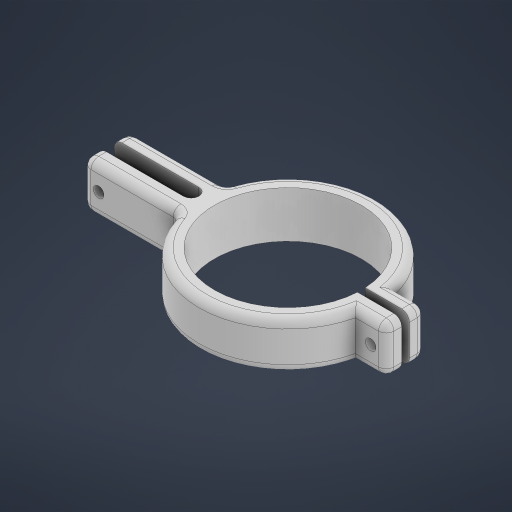
# Autodesk Inventor part: Clamp
Saved by Autodesk Inventor 2024.1 (Build 281209000, 209)
## iProperties
Created: 2024-11-18
Part Number: Clamp
Material: Generic
Document SubType Name: Modeling
Designer: Designer
Density: 1 g/cm^3
Appearance: Default
Author: Designer
Autodesk Inventor part; units mm, degrees
ref_plane "YZ Plane" through (0, 0, 0) normal (1, 0, 0) x (0, 1, 0)
ref_plane "XZ Plane" through (0, 0, 0) normal (0, 1, 0) x (-1, 0, 0)
ref_plane "XY Plane" through (0, 0, 0) normal (0, 0, 1) x (1, 0, 0)
sketch "Sketch1" plane through (0, 0, 0) normal (0, 1, 0) x (-1, 0, 0)
  line L0 (-22.0113, 1.5875) -> (-22.0113, 7.9375)
  line L1 (-22.0113, 7.9375) -> (-9.3113, 7.9375)
  arc A0 (-3.8366, -1.5875) -> (-3.8366, 1.5875) centre (26.2841, 0) ccw
  line L2 (-22.0113, 1.5875) -> (-8.3646, 1.5875)
  line L3 (-8.3646, -1.5875) -> (-22.0113, -1.5875)
  line L4 (-22.0113, -1.5875) -> (-22.0113, -7.9375)
  line L5 (-22.0113, -7.9375) -> (-9.3113, -7.9375)
  line L6 (61.4879, 9.525) -> (100.7583, 9.525)
  line L7 (100.7583, 9.525) -> (100.7583, 3.175)
  line L8 (100.7583, 3.175) -> (62.6583, 3.175)
  line L9 (62.6583, -3.175) -> (100.7583, -3.175)
  line L10 (100.7583, -3.175) -> (100.7583, -9.525)
  line L11 (100.7583, -9.525) -> (61.4879, -9.525)
  line L12 (-8.3646, 1.5875) -> (-3.8366, 1.5875)
  line L13 (-8.3646, -1.5875) -> (-3.8366, -1.5875)
  arc A1 (61.4879, 9.525) -> (-9.3113, 7.9375) centre (26.2841, 0) ccw
  arc A2 (-9.3113, -7.9375) -> (61.4879, -9.525) centre (26.2841, 0) ccw
  arc A3 (62.6583, -3.175) -> (62.6583, 3.175) centre (26.2841, 0) ccw
  point P0 (0, 0)
  dimension "d0" = 60.325
  dimension "d2" = 6.35
  dimension "d3" = 6.35
  dimension "d4" = 3.175
  dimension "d5" = 1.5875
  dimension "d6" = 6.35
  dimension "d7" = 6.35
  dimension "d8" = 6.35
  dimension "d9" = 3.175
  dimension "d10" = 6.35
  dimension "d11" = 38.1
  dimension "d12" = 12.7
  constraints: 28 end point, 8 point on circle, 6 perpendicular, 4 centre point, 4 horizontal, 3 parallel, 2 point on line, 1 coincident, 1 collinear, 1 concentric, 1 vertical
  measures "d0" diameter of A0
  measures "d2" distance of L3.end L4.end
  measures "d3" distance of L0.start L0.end
  measures "d4" distance between parallel lines of L2 L3
  measures "d5" distance from line of point (0, 0) L3
  measures "d6" distance between parallel lines of L9 L11
  measures "d7" distance between parallel lines of L6 L8
  measures "d8" distance between parallel lines of L8 L9
  measures "d9" distance from line of point (0, 0) L9
  measures "d10" radial gap between concentric circles of A0 A3
  measures "d11" distance of L7.end L8.end
  measures "d12" distance of L4.end L5.end
extrude "Extrusion1" add sketch "Sketch1" along normal blind 19.05
sketch "Sketch2" plane through (9.3113, 0, 7.9375) normal (0, 0, 1) x (1, 0, 0)
  circle A0 centre (6.35, 9.525) radius 2.1844
  line L0 (0, 19.05) -> (12.7, 19.05) projected
  line L1 (12.7, 0) -> (12.7, 19.05) projected
  circle A1 centre (-103.7196, 9.525) radius 2.1844
  line L2 (-110.0696, 0) -> (-110.0696, 19.05) projected
  line L3 (-110.0696, 19.05) -> (-70.7992, 19.05) projected
  point P0 (-9.3113, 0)
  dimension "d15" = 9.525
  dimension "d16" = 6.35
  dimension "d17" = 4.3688
  dimension "d18" = 6.35
  dimension "d19" = 9.525
  dimension "d20" = 4.3688
  constraints: 2 centre point
  measures "d15" distance from line of L0 A0.centre
  measures "d16" distance from line of L1 A0.centre
  measures "d17" diameter of A0
  measures "d18" distance from line of L2 A1.centre
  measures "d19" distance from line of L3 A1.centre
  measures "d20" diameter of A1
extrude "Extrusion2" cut sketch "Sketch2" along normal mid plane 50.8
fillet "Fillet1" radius 3.175 28 edges at (-81.1231, 19.05, 9.525) (-100.7583, 9.525, 9.525) (-81.1231, 0, 9.525) (-81.1231, 19.05, -9.525) (-100.7583, 9.525, -9.525) (-81.1231, 0, -9.525) (-61.4879, 9.525, -9.525) (-61.4879, 9.525, 9.525) (-62.6583, 9.525, -3.175) (-62.6583, 9.525, 3.175) (-25.4665, 19.05, -36.4605) (-25.4665, 0, -36.4605) (-25.4665, 19.05, 36.4605) (-25.4665, 0, 36.4605) (15.6613, 19.05, 7.9375) (22.0113, 9.525, 7.9375) (15.6613, 0, 7.9375) (15.6613, 19.05, -7.9375) (22.0113, 9.525, -7.9375) (15.6613, 0, -7.9375) (22.0113, 19.05, -4.7625) (22.0113, 19.05, 4.7625) (22.0113, 0, -4.7625) (22.0113, 0, 4.7625) (-100.7583, 19.05, -6.35) (-100.7583, 19.05, 6.35) (-100.7583, 0, -6.35) (-100.7583, 0, 6.35)
body "Solid1"
